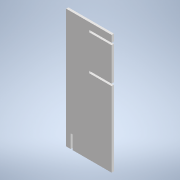
# Autodesk Inventor part: Stand
Saved by Autodesk Inventor 2020 (Build 240168000, 168)
## iProperties
Created: 2019-07-01
Part Number: Stand
Material: Generic
Document SubType Name: Modeling
Designer: eugen
Density: 1 g/cm^3
Appearance: Default
Author: eugen
Autodesk Inventor part; units mm, degrees
ref_plane "YZ Plane" through (0, 0, 0) normal (1, 0, 0) x (0, 1, 0)
ref_plane "XZ Plane" through (0, 0, 0) normal (0, 1, 0) x (-1, 0, 0)
ref_plane "XY Plane" through (0, 0, 0) normal (0, 0, 1) x (1, 0, 0)
sketch "Sketch1" plane through (0, 0, 0) normal (0, 0, 1) x (1, 0, 0)
  line L0 (0, 0) -> (127, 0)
  line L1 (127, 157.48) -> (127, 333.502)
  line L2 (127, 333.502) -> (0, 333.502)
  line L3 (0, 333.502) -> (0, 157.48)
  line L4 (64.77, 314.452) -> (127, 314.452)
  line L5 (127, 314.452) -> (127, 308.61)
  line L6 (127, 308.61) -> (64.77, 308.61)
  line L7 (63.5, 309.88) -> (63.5, 313.182)
  line L8 (64.77, 215.392) -> (127, 215.392)
  line L9 (127, 215.392) -> (127, 209.55)
  line L10 (127, 209.55) -> (64.77, 209.55)
  line L11 (63.5, 210.82) -> (63.5, 214.122)
  line L12 (127, 208.28) -> (127, 202.438)
  line L13 (0, 152.4) -> (127, 152.4) construction
  line L14 (0, 157.48) -> (0, 0)
  line L15 (127, 157.48) -> (127, 0)
  line L16 (12.7, 0) -> (18.542, 0)
  line L17 (18.542, 0) -> (18.542, 36.83)
  line L18 (17.272, 38.1) -> (13.97, 38.1)
  line L19 (12.7, 36.83) -> (12.7, 0)
  arc A0 (64.77, 314.452) -> (63.5, 313.182) centre (64.77, 313.182) ccw
  arc A1 (63.5, 309.88) -> (64.77, 308.61) centre (64.77, 309.88) ccw
  arc A2 (64.77, 215.392) -> (63.5, 214.122) centre (64.77, 214.122) ccw
  arc A3 (63.5, 210.82) -> (64.77, 209.55) centre (64.77, 210.82) ccw
  arc A4 (18.542, 36.83) -> (17.272, 38.1) centre (17.272, 36.83) ccw
  arc A5 (13.97, 38.1) -> (12.7, 36.83) centre (13.97, 36.83) ccw
  point P0 (63.5, 314.452)
  point P1 (63.5, 308.61)
  point P2 (63.5, 215.392)
  point P3 (63.5, 209.55)
  point P4 (127, 209.55)
  point P5 (127, 215.392)
  point P6 (127, 308.61)
  point P7 (127, 314.452)
  point P8 (18.542, 38.1)
  point P9 (12.7, 38.1)
  point P10 (127, 152.4)
  dimension "d1" = 5.842
  dimension "d7" = 127
  dimension "d8" = 5.842
  dimension "d27" = 152.4
  dimension "d30" = 99.06
  dimension "d32" = 19.05
  dimension "d33" = 63.5
  dimension "d34" = 5.842
  dimension "d35" = 12.7
  dimension "d36" = 38.1
  dimension "d37" = 209.55
  dimension "d38" = 1.27
  dimension "d39" = 1.27
  dimension "d40" = 1.27
  constraints: 40 end point, 16 point on line, 12 point on circle, 12 tangent, 8 parallel, 6 centre point, 5 collinear, 5 horizontal, 4 perpendicular, 3 equal radius, 2 vertical
  measures "d1" distance of L4.end L5.end
  measures "d7" distance between parallel lines of L1 L3
  measures "d8" distance of L8.end L9.end
  measures "d27" distance from line of L0 L13.start
  measures "d30" distance between parallel lines of L10 L6
  measures "d32" distance between parallel lines of L2 L4
  measures "d33" distance between parallel lines of L3 L11
  measures "d34" distance of point (18.542, 38.1) point (12.7, 38.1)
  measures "d35" distance between parallel lines of L14 L19
  measures "d36" distance between parallel lines of L0 L18
  measures "d37" distance between parallel lines of L10 L0
  measures "d38" radius of A0
  measures "d39" radius of A1
  measures "d40" radius of A4
extrude "Extrusion1" add sketch "Sketch1" along normal blind 6.35 contours L14 L3 L2 L1 L4 A0 L7 A1 L6 L8 A2 L11 A3 L10 L15 L0 L17 A4 L18 A5 L19
equation "\"d33\" = 0.5 * d7"
body "Solid1"
